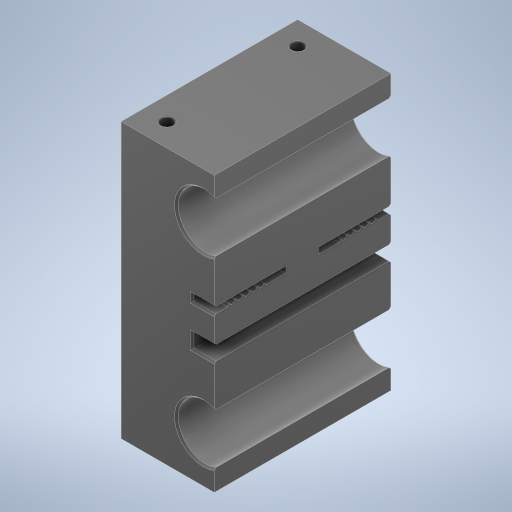
# Autodesk Inventor part: Carriage Design Left
Saved by Autodesk Inventor 2023 (Build 270158000, 158)
## iProperties
Created: 2023-02-06
Part Number: Carriage Design Left
Material: Generic
Document SubType Name: Modeling
Designer: mbear
Density: 1 g/cm^3
Appearance: Smooth - Black
Author: mbear
## iProperties of the stored document Carriage Design Left_3DPrint.ipt
Created: 2023-02-13
Part Number: Carriage Design Left_3DPrint
Material: Generic
Document SubType Name: Modeling
Designer: mbear
Density: 1 g/cm^3
Appearance: Default
Author: mbear
Autodesk Inventor part; units mm, degrees
ref_plane "XZ Plane" through (0, 0, 0) normal (0, 1, 0) x (-1, 0, 0)
ref_plane "XY Plane" through (0, 0, 0) normal (0, 0, 1) x (1, 0, 0)
sketch "Sketch1" plane through (0, 0, 0) normal (0, 0, 1) x (1, 0, 0)
  line L0 (-22.86, 0) -> (22.86, 0)
  line L1 (22.86, 0) -> (22.86, 76.2)
  line L2 (22.86, 76.2) -> (-22.86, 76.2)
  line L3 (-22.86, 76.2) -> (-22.86, 0)
  circle A0 centre (0, 63.5) radius 7.5635
  circle A1 centre (0, 12.7) radius 7.5635
  point P0 (0, 0)
  point P1 (0, 76.2)
  point P2 (0, 0)
  dimension "d0" = 76.2
  dimension "d1" = 15.127
  dimension "d2" = 15.127
  dimension "d3" = 45.72
  dimension "d4" = 12.7
  dimension "d5" = 50.8
  dimension "d7" = 12.7
  dimension "d8" = 0
  constraints: 8 end point, 4 vertical alignment, 2 centre point, 2 midpoint, 2 parallel, 1 horizontal, 1 perpendicular
  measures "d0" distance between parallel lines of L0 L2
  measures "d1" diameter of A0
  measures "d2" diameter of A1
  measures "d3" distance between parallel lines of L1 L3
  measures "d4" distance from line of L2 A0.centre
  measures "d5" distance of A1.centre A0.centre
  measures "d7" distance from line of L0 A1.centre
  measures "d8" distance from line of point (0, 0) L0
extrude "Extrusion1" add sketch "Sketch1" along normal blind 49
chamfer "Chamfer1" distance 0.508 angle 45 4 edges at (-7.5635, 63.5, 49) (-7.5635, 12.7, 49) (-7.5635, 63.5, 0) (-7.5635, 12.7, 0)
ref_plane "Work Plane2" through (3, 0, 0) normal (1, 0, 0) x (0, 1, 0)
ref_plane "Work Plane1" through (0, 0, 0) normal (1, 0, 0) x (0, 1, 0)
sketch "Sketch4" plane through (3, 0, 0) normal (1, 0, 0) x (0, 1, 0)
  line L0 (81.7933, 51.2911) -> (-4.404, 51.2911)
  line L1 (-4.404, 51.2911) -> (-4.404, -2.2911)
  line L2 (-4.404, -2.2911) -> (81.7933, -2.2911)
  line L3 (81.7933, -2.2911) -> (81.7933, 51.2911)
  point P0 (0, 0)
  constraints: 8 end point, 2 parallel, 1 horizontal, 1 perpendicular
extrude "Extrusion3" cut sketch "Sketch4" along normal blind 25.4
sketch "Sketch5" plane through (3, 0, 0) normal (1, 0, 0) x (0, 0, -1)
  line L0 (-49, 44.1724) -> (-29, 44.1724)
  line L1 (-29, 44.1724) -> (-29, 42.6484)
  line L2 (-44.8559, 43.4084) -> (-49, 43.4084)
  line L3 (-29, 42.6484) -> (-32, 42.6484)
  line L4 (-32, 44.1724) -> (-32, 42.6484)
  line L5 (-34, 44.1724) -> (-34, 42.6484)
  line L6 (-36, 44.1724) -> (-36, 42.6484)
  line L7 (-38, 44.1724) -> (-38, 42.6484)
  line L8 (-40, 44.1724) -> (-40, 42.6484)
  line L9 (-42, 44.1724) -> (-42, 42.6484)
  line L10 (-44, 44.1724) -> (-44, 42.6484)
  arc A0 (-44, 42.6484) -> (-43.2434, 43.32) centre (-44, 43.4104) ccw
  arc A1 (-42.7566, 43.32) -> (-42, 42.6484) centre (-42, 43.4104) ccw
  arc A2 (-42, 42.6484) -> (-41.2434, 43.32) centre (-42, 43.4104) ccw
  arc A3 (-44.7566, 43.3202) -> (-44, 42.6484) centre (-44, 43.4104) ccw
  arc A4 (-40.7566, 43.32) -> (-40, 42.6484) centre (-40, 43.4104) ccw
  arc A5 (-40, 42.6484) -> (-39.2434, 43.3202) centre (-40, 43.4104) ccw
  arc A6 (-38.7566, 43.3202) -> (-38, 42.6484) centre (-38, 43.4104) ccw
  arc A7 (-38, 42.6484) -> (-37.2434, 43.3202) centre (-38, 43.4104) ccw
  arc A8 (-36.7566, 43.3202) -> (-36, 42.6484) centre (-36, 43.4104) ccw
  arc A9 (-36, 42.6484) -> (-35.2433, 43.3204) centre (-36, 43.4104) ccw
  line L11 (-32, 42.6484) -> (-49, 42.6484)
  arc A10 (-44.7566, 43.3202) -> (-44.8421, 43.4074) centre (-44.8559, 43.3084) ccw
  line L12 (-43.1441, 43.4081) -> (-42.8559, 43.4081)
  line L13 (-41.1441, 43.4081) -> (-40.8559, 43.4081)
  line L14 (-39.1441, 43.4084) -> (-38.8559, 43.4084)
  line L15 (-37.1441, 43.4084) -> (-36.8559, 43.4084)
  line L16 (-35.1442, 43.4086) -> (-34, 43.4104)
  arc A11 (-43.1441, 43.4081) -> (-43.2434, 43.32) centre (-43.1441, 43.3081) ccw
  arc A12 (-42.7566, 43.32) -> (-42.8559, 43.4081) centre (-42.8559, 43.3081) ccw
  arc A13 (-41.1441, 43.4081) -> (-41.2434, 43.32) centre (-41.1441, 43.3081) ccw
  arc A14 (-40.7566, 43.32) -> (-40.8559, 43.4081) centre (-40.8559, 43.3081) ccw
  arc A15 (-39.1441, 43.4084) -> (-39.2434, 43.3202) centre (-39.1441, 43.3084) ccw
  arc A16 (-38.7566, 43.3202) -> (-38.8559, 43.4084) centre (-38.8559, 43.3084) ccw
  arc A17 (-37.1441, 43.4084) -> (-37.2434, 43.3202) centre (-37.1441, 43.3084) ccw
  arc A18 (-36.7566, 43.3202) -> (-36.8559, 43.4084) centre (-36.8559, 43.3084) ccw
  arc A19 (-35.1581, 43.4076) -> (-35.2433, 43.3204) centre (-35.144, 43.3086) ccw
  line L17 (-35.1442, 43.4086) -> (-35.1442, 42.6484)
  line L18 (-44.8622, 43.3976) -> (-45.2947, 42.6484)
  arc A20 (-44.8421, 43.4074) -> (-44.8622, 43.3976) centre (-44.8448, 43.3876) ccw
  line L19 (-35.138, 43.3978) -> (-34.7037, 42.6484)
  arc A21 (-35.138, 43.3978) -> (-35.1581, 43.4076) centre (-35.1553, 43.3878) ccw
  line L20 (-29, 44.1724) -> (-49, 44.1724)
  line L21 (-49, 44.1724) -> (-49, 44.4724)
  line L22 (-49, 44.4724) -> (-29, 44.4724)
  line L23 (-29, 44.4724) -> (-29, 44.1724)
  line L24 (-48.492, 56.5569) -> (-0.508, 56.5569) projected
  line L25 (-49, 76.2) -> (-49, 0) projected
  line L26 (0, 38.0485) -> (0, 34.0485)
  line L27 (0, 76.2) -> (0, 70.9933) projected
  line L28 (0, 76.2) -> (-49, 76.2) projected
  line L29 (-24.5, 76.2) -> (-24.5, 0)
  line L30 (0, 0) -> (-49, 0) projected
  line L31 (0, 44.1724) -> (-20, 44.1724)
  line L32 (-20, 44.1724) -> (-20, 42.6484)
  line L33 (-4.1441, 43.4084) -> (0, 43.4084)
  line L34 (-20, 42.6484) -> (-17, 42.6484)
  line L35 (-17, 44.1724) -> (-17, 42.6484)
  line L36 (-15, 44.1724) -> (-15, 42.6484)
  line L37 (-13, 44.1724) -> (-13, 42.6484)
  line L38 (-11, 44.1724) -> (-11, 42.6484)
  line L39 (-9, 44.1724) -> (-9, 42.6484)
  line L40 (-7, 44.1724) -> (-7, 42.6484)
  line L41 (-5, 44.1724) -> (-5, 42.6484)
  arc A22 (-5.7566, 43.32) -> (-5, 42.6484) centre (-5, 43.4104) ccw
  arc A23 (-7, 42.6484) -> (-6.2434, 43.32) centre (-7, 43.4104) ccw
  arc A24 (-7.7566, 43.32) -> (-7, 42.6484) centre (-7, 43.4104) ccw
  arc A25 (-5, 42.6484) -> (-4.2434, 43.3202) centre (-5, 43.4104) ccw
  arc A26 (-9, 42.6484) -> (-8.2434, 43.32) centre (-9, 43.4104) ccw
  arc A27 (-9.7566, 43.3202) -> (-9, 42.6484) centre (-9, 43.4104) ccw
  arc A28 (-11, 42.6484) -> (-10.2434, 43.3202) centre (-11, 43.4104) ccw
  arc A29 (-11.7566, 43.3202) -> (-11, 42.6484) centre (-11, 43.4104) ccw
  arc A30 (-13, 42.6484) -> (-12.2434, 43.3202) centre (-13, 43.4104) ccw
  arc A31 (-13.7567, 43.3204) -> (-13, 42.6484) centre (-13, 43.4104) ccw
  line L42 (-17, 42.6484) -> (0, 42.6484)
  arc A32 (-4.1579, 43.4074) -> (-4.2434, 43.3202) centre (-4.1441, 43.3084) ccw
  line L43 (-5.8559, 43.4081) -> (-6.1441, 43.4081)
  line L44 (-7.8559, 43.4081) -> (-8.1441, 43.4081)
  line L45 (-9.8559, 43.4084) -> (-10.1441, 43.4084)
  line L46 (-11.8559, 43.4084) -> (-12.1441, 43.4084)
  line L47 (-13.8558, 43.4086) -> (-15, 43.4104)
  arc A33 (-5.7566, 43.32) -> (-5.8559, 43.4081) centre (-5.8559, 43.3081) ccw
  arc A34 (-6.1441, 43.4081) -> (-6.2434, 43.32) centre (-6.1441, 43.3081) ccw
  arc A35 (-7.7566, 43.32) -> (-7.8559, 43.4081) centre (-7.8559, 43.3081) ccw
  arc A36 (-8.1441, 43.4081) -> (-8.2434, 43.32) centre (-8.1441, 43.3081) ccw
  arc A37 (-9.7566, 43.3202) -> (-9.8559, 43.4084) centre (-9.8559, 43.3084) ccw
  arc A38 (-10.1441, 43.4084) -> (-10.2434, 43.3202) centre (-10.1441, 43.3084) ccw
  arc A39 (-11.7566, 43.3202) -> (-11.8559, 43.4084) centre (-11.8559, 43.3084) ccw
  arc A40 (-12.1441, 43.4084) -> (-12.2434, 43.3202) centre (-12.1441, 43.3084) ccw
  arc A41 (-13.7567, 43.3204) -> (-13.8419, 43.4076) centre (-13.856, 43.3086) ccw
  line L48 (-13.8558, 43.4086) -> (-13.8558, 42.6484)
  line L49 (-4.1378, 43.3976) -> (-3.7053, 42.6484)
  arc A42 (-4.1378, 43.3976) -> (-4.1579, 43.4074) centre (-4.1552, 43.3876) ccw
  line L50 (-13.862, 43.3978) -> (-14.2963, 42.6484)
  arc A43 (-13.8419, 43.4076) -> (-13.862, 43.3978) centre (-13.8447, 43.3878) ccw
  line L51 (-20, 44.1724) -> (0, 44.1724)
  line L52 (0, 44.1724) -> (0, 44.4724)
  line L53 (0, 44.4724) -> (-20, 44.4724)
  line L54 (-20, 44.4724) -> (-20, 44.1724)
  line L55 (0, 44.1724) -> (0, 42.6484)
  line L56 (0, 76.2) -> (0, 0) projected
  line L57 (-4.1441, 43.4084) -> (-4.1464, 43.4056)
  point P0 (-43.34, 43.4084)
  point P1 (-42.66, 43.4084)
  point P2 (-43.238, 43.4081)
  point P3 (-42.762, 43.4081)
  point P4 (-41.34, 43.4084)
  point P5 (-40.66, 43.4084)
  point P6 (-39.34, 43.4084)
  point P7 (-38.66, 43.4084)
  point P8 (-37.34, 43.4084)
  point P9 (-36.66, 43.4084)
  point P10 (-35.34, 43.4084)
  point P11 (-34.66, 43.4084)
  point P12 (-33.34, 43.4084)
  point P13 (-32.66, 43.4084)
  point P14 (-32, 43.4104)
  point P15 (-41.238, 43.4081)
  point P16 (-44.762, 43.4084)
  point P17 (-40.762, 43.4081)
  point P18 (-39.238, 43.4084)
  point P19 (-38.762, 43.4084)
  point P20 (-37.238, 43.4084)
  point P21 (-36.762, 43.4084)
  point P22 (-35.238, 43.4084)
  point P23 (0, 73.5966)
  point P24 (-5.66, 43.4084)
  point P25 (-6.34, 43.4084)
  point P26 (-5.762, 43.4081)
  point P27 (-6.238, 43.4081)
  point P28 (-7.66, 43.4084)
  point P29 (-8.34, 43.4084)
  point P30 (-9.66, 43.4084)
  point P31 (-10.34, 43.4084)
  point P32 (-11.66, 43.4084)
  point P33 (-12.34, 43.4084)
  point P34 (-13.66, 43.4084)
  point P35 (-14.34, 43.4084)
  point P36 (-15.66, 43.4084)
  point P37 (-16.34, 43.4084)
  point P38 (-17, 43.4104)
  point P39 (-7.762, 43.4081)
  point P40 (-4.238, 43.4084)
  point P41 (-8.238, 43.4081)
  point P42 (-9.762, 43.4084)
  point P43 (-10.238, 43.4084)
  point P44 (-11.762, 43.4084)
  point P45 (-12.238, 43.4084)
  point P46 (-13.762, 43.4084)
  point P47 (-36, 42.6484)
  point P48 (-36, 42.6484)
  dimension "d29" = 20
  dimension "d30" = 1.524
  dimension "d32" = 0.76
  dimension "d33" = 3
  dimension "d34" = 2
  dimension "d35" = 2
  dimension "d36" = 2
  dimension "d37" = 2
  dimension "d38" = 2
  dimension "d39" = 2
  dimension "d40" = 0.66
  dimension "d41" = 0.66
  dimension "d43" = 0.66
  dimension "d44" = 0.66
  dimension "d45" = 0.66
  dimension "d46" = 0.66
  dimension "d47" = 0.66
  dimension "d48" = 0.66
  dimension "d49" = 0.66
  dimension "d50" = 0.66
  dimension "d51" = 0.66
  dimension "d52" = 0.66
  dimension "d53" = 0.1
  dimension "d54" = 0.1
  dimension "d55" = 60
  dimension "d56" = 0.02
  dimension "d57" = 60
  dimension "d58" = 0.02
  dimension "d61" = 0.3
  dimension "d63" = 12.0845
  dimension "d66" = 49
  constraints: 123 point on circle, 100 symmetric about line, 96 end point, 44 centre point, 30 point on line, 23 tangent, 16 coincident, 10 midpoint, 8 equal radius, 8 vertical, 4 parallel, 3 horizontal, 2 collinear, 2 horizontal alignment, 2 perpendicular, 82 other
  measures "d29" distance of point (-49, 44.172) L1.start
  measures "d30" distance of L1.start L1.end
  measures "d33" distance from line of L1 L3.end
  measures "d34" distance between parallel lines of L4 L5
  measures "d35" distance between parallel lines of L5 L6
  measures "d36" distance between parallel lines of L6 L7
  measures "d37" distance between parallel lines of L7 L8
  measures "d38" distance between parallel lines of L8 L9
  measures "d39" distance between parallel lines of L10 L9
  measures "d40" distance from line of point (-43.34, 43.408) L10
  measures "d41" horizontal distance of L9.end point (-42.66, 43.408)
  measures "d43" distance of point (-41.34, 43.408) A1.centre
  measures "d44" distance of point (-40, 43.41) point (-40.66, 43.408)
  measures "d45" distance of point (-39.34, 43.408) point (-40, 43.41)
  measures "d46" distance of point (-38, 43.41) point (-38.66, 43.408)
  measures "d47" distance of point (-37.34, 43.408) point (-38, 43.41)
  measures "d48" distance of point (-36, 43.41) point (-36.66, 43.408)
  measures "d49" distance of point (-35.34, 43.408) point (-36, 43.41)
  measures "d50" distance of L16.end point (-34.66, 43.408)
  measures "d51" distance of point (-33.34, 43.408) L16.end
  measures "d52" distance of point (-32, 43.41) point (-32.66, 43.408)
  measures "d53" radius of A10
  measures "d54" radius of A11
  measures "d55" angle to the sketch x axis of L18
  measures "d56" radius of A20
  measures "d57" angle of L16 L19
  measures "d58" radius of A21
  measures "d63" distance between parallel lines of L22 L24
  measures "d66" distance from line of point (0, 73.597) L25
extrude "Extrusion4" cut sketch "Sketch5" against normal blind 6.2 contours L21 L22 L23 L0 | L0 L10 A3 A10 A20 L18 L11 L25 | L0 L9 A1 A12 L12 A11 A0 L10 | L0 L8 A4 A14 L13 A13 A2 L9 | L0 L7 A6 A16 L14 A15 A5 L8 | L1 L3 L4 L0 | L0 L6 A8 A18 L15 A17 A7 L7 | L4 L11 L5 L0 | L0 L5 L16 L17 A21 A19 A9 L6 | L5 L11 L19 A21 L17 L16 | L52 L31 L54 L53 | L55 L33 L57 A42 A32 A25 L41 L31 | L41 A22 A33 L43 A34 A23 L40 L31 | L55 L42 L49 A42 L57 L33 | L31 L35 L34 L32 | L40 A24 A35 L44 A36 A26 L39 L31 | L31 L36 L42 L35 | L39 A27 A37 L45 A38 A28 L38 L31 | L31 L37 A31 A41 A43 L48 L47 L36 | L38 A29 A39 L46 A40 A30 L37 L31 | L47 L48 A43 L50 L42 L36
fillet "Fillet1" radius 0.2 4 edges at (-0.1, 42.6484, 45.2947) (-0.1, 42.6484, 34.7037) (-0.1, 44.4724, 29) (-0.1, 42.6484, 29)
fillet "Fillet2" radius 0.2 4 edges at (-0.1, 42.6484, 3.7053) (-0.1, 42.6484, 14.2963) (-0.1, 42.6484, 20) (-0.1, 44.4724, 20)
chamfer "Chamfer2" distance 0.5 angle 45 6 edges at (-0.1, 44.4724, 0) (-3.2, 43.5604, 0) (-0.1, 42.6484, 0) (-3.2, 43.5604, 49) (-0.1, 44.4724, 49) (-0.1, 42.6484, 49)
sketch "Sketch7" plane through (3, 0, 0) normal (1, 0, 0) x (0, 0, -1)
  line L0 (-49, 76.2) -> (-49, 0) projected
  line L1 (-49, 33.2923) -> (0, 33.2923)
  arc A0 (-29.2, 42.6484) -> (-29, 42.8484) centre (-29.2, 42.8484) ccw projected
  line L2 (0, 42.1484) -> (0, 20.1933) projected
  line L3 (-49, 35.2923) -> (0, 35.2923)
  line L4 (0, 35.2923) -> (0, 31.2923)
  line L5 (0, 31.2923) -> (-49, 31.2923)
  line L6 (-49, 31.2923) -> (-49, 35.2923)
  point P0 (0, 0)
  point P1 (-29.0586, 42.707)
  point P2 (0, 35.2923)
  point P3 (-49, 31.2923)
  dimension "d71" = 9.4147
  dimension "d72" = 4
  dimension "d73" = 2
  constraints: 10 end point, 3 point on line, 2 horizontal, 2 parallel, 1 perpendicular, 1 point on circle
  measures "d71" distance from line of L1 point (-29.059, 42.707)
  measures "d72" distance between parallel lines of L5 L3
  measures "d73" distance between parallel lines of L1 L3
extrude "Extrusion5" cut sketch "Sketch7" against normal blind 6.2
chamfer "Chamfer3" distance 0.5 angle 45 6 edges at (-0.1, 35.2923, 0) (-3.2, 33.2923, 0) (-0.1, 31.2923, 0) (-0.1, 31.2923, 49) (-3.2, 33.2923, 49) (-0.1, 35.2923, 49)
sketch "Sketch8" plane through (-22.86, 76.2, 49) normal (0, 1, 0) x (1, 0, 0)
  circle A0 centre (6.35, 42.65) radius 2.0172
  circle A1 centre (6.35, 6.35) radius 2.0563
  line L0 (0, 49) -> (0, 0) projected
  line L1 (25.86, 49) -> (0, 49) projected
  line L2 (25.86, 0) -> (0, 0) projected
  point P0 (22.86, 49)
  dimension "d79" = 4.0344
  dimension "d80" = 6.35
  dimension "d81" = 6.35
  dimension "d82" = 6.35
  dimension "d83" = 6.35
  constraints: 2 centre point
  measures "d79" diameter of A0
  measures "d80" distance from line of L0 A0.centre
  measures "d81" distance from line of L1 A0.centre
  measures "d82" distance from line of A1.centre L0
  measures "d83" distance from line of L2 A1.centre
hole "Hole1" at (-16.51, 76.2, 6.35) at (-16.51, 76.2, 42.65) direction (0, -1, 0) diameter 3.4 depth 10 tip angle 118 clearance for "Socket Head Cap Screw" size "M3" standard "Ansi Metric M Profile"
fillet "Fillet3" radius 0.2 2 edges at (-16.51, 76.2, 4.65) (-16.51, 76.2, 40.95)
sketch "Sketch9" plane through (-22.86, 0, 0) normal (-1, 0, 0) x (0, 0, 1)
  line L0 (4.65, 76) -> (8.05, 76) projected
  line L1 (40.95, 76) -> (44.35, 76) projected
  line L2 (6.35, 76) -> (6.35, 0)
  line L3 (2.35, 69.2) -> (10.35, 69.2)
  line L4 (10.35, 69.2) -> (10.35, 66.7)
  line L5 (10.35, 66.7) -> (2.35, 66.7)
  line L6 (2.35, 66.7) -> (2.35, 69.2)
  line L7 (6.35, 69.2) -> (6.35, 69.2)
  line L8 (6.35, 69.2) -> (6.35, 74.5973)
  line L9 (6.35, 74.5973) -> (6.35, 74.5973)
  line L10 (6.35, 74.5973) -> (6.35, 69.2)
  line L11 (49, 76.2) -> (0, 76.2) projected
  line L12 (24.5, 76.2) -> (24.5, 0)
  line L13 (0, 0) -> (49, 0) projected
  line L14 (46.65, 69.2) -> (38.65, 69.2)
  line L15 (38.65, 69.2) -> (38.65, 66.7)
  line L16 (38.65, 66.7) -> (46.65, 66.7)
  line L17 (46.65, 66.7) -> (46.65, 69.2)
  point P0 (10.35, 67.95)
  point P1 (2.35, 67.95)
  dimension "d92" = 8
  dimension "d93" = 2.5
  dimension "d94" = 7
  constraints: 28 end point, 6 midpoint, 4 equal length, 4 symmetric about line, 2 horizontal, 2 perpendicular, 1 point on line, 1 vertical, 1 vertical alignment
  measures "d92" distance of point (10.35, 67.95) point (2.35, 67.95)
  measures "d93" distance between parallel lines of L5 L3
  measures "d94" distance between parallel lines of L3 L11
extrude "Extrusion6" cut sketch "Sketch9" against normal blind 13.35
fillet "Fillet4" radius 0.2 4 edges at (-16.51, 66.7, 40.95) (-16.51, 66.7, 4.65) (-16.51, 69.2, 40.95) (-16.51, 69.2, 4.65)
chamfer "Chamfer4" distance 0.5 angle 45 8 edges at (-22.86, 69.2, 6.35) (-22.86, 67.95, 10.35) (-22.86, 66.7, 6.35) (-22.86, 67.95, 2.35) (-22.86, 69.2, 42.65) (-22.86, 67.95, 38.65) (-22.86, 66.7, 42.65) (-22.86, 67.95, 46.65)
equation "\"d1\" = d2"
body "Solid1"
